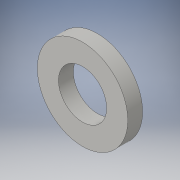
# Autodesk Inventor part: washer_m3_r01
Saved by Autodesk Inventor 2016 (Build 200138000, 138)
## iProperties
Created: 2017-01-09
Part Number: washer_m3_r01
Material: Generic
Document SubType Name: Modeling
Designer: Valued Customer
Density: 1 g/cm^3
Appearance: Default
Author: Valued Customer
Autodesk Inventor part; units mm, degrees
ref_plane "YZ Plane" through (0, 0, 0) normal (1, 0, 0) x (0, 1, 0)
ref_plane "XZ Plane" through (0, 0, 0) normal (0, 1, 0) x (-1, 0, 0)
ref_plane "XY Plane" through (0, 0, 0) normal (0, 0, 1) x (1, 0, 0)
sketch "Sketch1" plane through (0, 0, 0) normal (0, 0, 1) x (1, 0, 0)
  circle A0 centre (0, 0) radius 3.048
  circle A1 centre (0, 0) radius 1.625
  dimension "d0" = 6.096
  dimension "d1" = 3.25
  constraints: 2 centre point, 2 coincident
  measures "d0" diameter of A0
  measures "d1" diameter of A1
extrude "Extrusion1" add sketch "Sketch1" along normal blind 1
body "Solid1"
